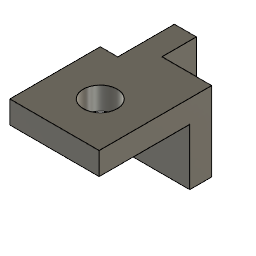
Button_Holder (Autodesk Fusion 360 design; units mm, degrees)
Autodesk Fusion 360 part; units mm, degrees
sketch "Sketch1" plane through (0, 0, 0) normal (0, 0, 1) x (1, 0, 0)
  line L0 (0, 0) -> (6.35, 0)
  line L1 (6.35, 0) -> (6.35, 1.95)
  line L2 (6.35, 1.95) -> (1.95, 1.95)
  line L3 (0, 4.3112) -> (0, 0)
  line L4 (0, 0) -> (5, 0)
  line L5 (1.95, 1.95) -> (1.95, 5)
  line L6 (1.95, 5) -> (0, 5)
  line L7 (0, 5) -> (0, 0)
  dimension "d1" = 1.95
  dimension "d2" = 1.95
  dimension "d5" = 4.4
  dimension "d6" = 3.05
  constraint horizontal L0
  constraint vertical L1
  constraint horizontal L2
  constraint vertical L3
  constraint coincident L0.start L3.end
  constraint horizontal L4
  constraint vertical L5
  constraint horizontal L6
  constraint vertical L7
  measures "d1" distance of L5.end L6.end
  measures "d2" distance of L0 L2
  measures "d5" distance of L1.end L2.end
  measures "d6" distance of L5.end L2.end
extrude "Extrude1" add sketch "Sketch1" along normal blind 7
sketch "Sketch2" plane through (0, 0, 0) normal (0, -1, 0) x (1, 0, 0)
  line L0 (0, 0) -> (6.35, 0)
  line L1 (6.35, 0) -> (6.35, 7)
  line L2 (6.35, 7) -> (0, 7)
  line L3 (0, 7) -> (0, 0)
  line L4 (6.35, 7) -> (-1.55, 7)
  line L5 (-1.55, 7) -> (-1.55, 5)
  line L6 (-1.55, 5) -> (6.35, 5)
  line L7 (6.35, 5) -> (6.35, 7)
  dimension "d9" = 2
  dimension "d10" = 7.9
  constraint horizontal L4
  constraint vertical L5
  constraint horizontal L6
  constraint vertical L7
  constraint collinear L1 L7
  constraint collinear L2 L4
  measures "d9" distance of L4.end L5.end
  measures "d10" distance of L1.end L4.end
extrude "Extrude2" add sketch "Sketch2" along normal blind 8 contours L3 L4 L5 L6 | L1 L2 L3 L4 L6 L7
sketch "Sketch3" plane through (0, 0, 7) normal (0, 0, 1) x (-1, 0, 0)
  line L0 (0, -5) -> (0, 0)
  line L1 (0, 0) -> (1.55, 0)
  line L2 (1.55, 0) -> (1.55, 8)
  line L3 (1.55, 8) -> (-6.35, 8)
  line L4 (-6.35, 8) -> (-6.35, -1.95)
  line L5 (-6.35, -1.95) -> (-1.95, -1.95)
  line L6 (-1.95, -1.95) -> (-1.95, -5)
  line L7 (-1.95, -5) -> (0, -5)
  circle A0 centre (-2.45, 4) radius 1.5
  dimension "d14" = 4
  dimension "d15" = 4
  dimension "d16" = 3
  measures "d14" distance of L3 A0.centre
  measures "d15" distance of L2 A0.centre
  measures "d16" diameter of A0
extrude "Extrude3" cut sketch "Sketch3" against normal blind 4 contours A0
